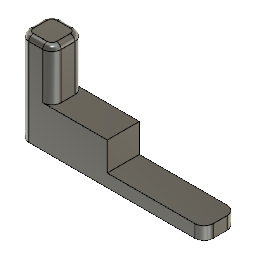
t-nut raiser v6 (Autodesk Fusion 360 design; units mm, degrees)
Autodesk Fusion 360 part; units mm, degrees
sketch "Sketch1" plane through (0, 0, 0) normal (0, 0, 1) x (1, 0, 0)
  line L0 (0, 3.5) -> (40, 3.5)
  line L1 (40, 3.5) -> (40, -3.5)
  line L2 (40, -3.5) -> (0, -3.5)
  line L3 (0, -3.5) -> (0, 3.5)
  line L4 (0, 3.5) -> (7, 3.5)
  line L5 (7, 3.5) -> (7, -3.5)
  line L6 (7, -3.5) -> (0, -3.5)
  line L7 (0, -3.5) -> (0, 3.5)
  line L8 (40, 3.5) -> (19, 3.5)
  line L9 (19, 3.5) -> (19, -3.5)
  line L10 (19, -3.5) -> (40, -3.5)
  line L11 (40, -3.5) -> (40, 3.5)
  dimension "d1" = 7
  dimension "d2" = 40
  dimension "d5" = 7
  dimension "d14" = 21
  dimension "d19" = 34
  constraint horizontal L0
  constraint vertical L1
  constraint horizontal L2
  constraint vertical L3
  constraint midpoint origin L3
  constraint horizontal L4
  constraint vertical L5
  constraint horizontal L6
  constraint vertical L7
  constraint midpoint origin L7
  constraint collinear L2 L6
  constraint horizontal L8
  constraint vertical L9
  constraint horizontal L10
  constraint vertical L11
  measures "d1" distance of L0.start L2.end
  measures "d2" distance of L1.end L2.end
  measures "d5" distance of L0.start L4.end
  measures "d14" distance of L0.end L8.end
extrude "Extrude3" add sketch "Sketch1" along normal blind 9 contours L0 L2 L5 L9 makes body 1
extrude "Extrude2" add sketch "Sketch1" along normal blind 20 separate body contours L0 L2 L3 L4 L5 L6 L7 makes body 2
extrude "Extrude1" add sketch "Sketch1" along normal blind 2.8 bodies 1 2
fillet "Fillet3" radius 2 6 edges at (7, -3.5, 14.5) (0, -3.5, 10) (0, 3.5, 10) (7, 3.5, 14.5) (40, 3.5, 1.4) (40, -3.5, 1.4) on bodies 1
fillet "Fillet4" radius 1 8 edges at (6.4142, -2.9142, 20) (7, 0, 20) (6.4142, 2.9142, 20) (3.5, 3.5, 20) (0.5858, 2.9142, 20) (0, 0, 20) (0.5858, -2.9142, 20) (3.5, -3.5, 20) on bodies 1
